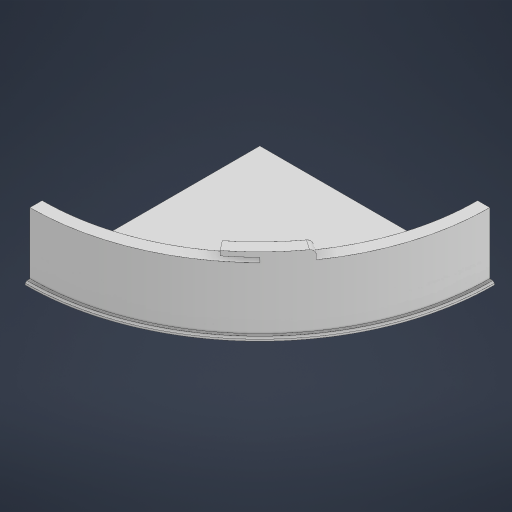
# Autodesk Inventor part: Head_Quad_V1
Saved by Autodesk Inventor 2024 (Build 280153000, 153)
## iProperties
Created: 2025-09-10
Part Number: Head_Quad_V1
Material: Generic
Document SubType Name: Modeling
Designer: kevin
Density: 1 g/cm^3
Appearance: Default
Author: kevin
Autodesk Inventor part; units mm, degrees
ref_plane "YZ Plane" through (0, 0, 0) normal (1, 0, 0) x (0, 1, 0)
ref_plane "XZ Plane" through (0, 0, 0) normal (0, 1, 0) x (-1, 0, 0)
ref_plane "XY Plane" through (0, 0, 0) normal (0, 0, 1) x (1, 0, 0)
sketch "Sketch1" plane through (0, 0, 0) normal (0, 1, 0) x (-1, 0, 0)
  arc A0 (0, 152.4) -> (-152.4, 0) centre (0, 0) ccw
  arc A1 (0, 149.4) -> (-149.4, 0) centre (0, 0) ccw
  line L0 (0, 152.4) -> (0, 0)
  line L1 (0, 152.4) -> (0, 0)
  line L2 (0, 0) -> (-152.4, 0)
  dimension "d0" = 304.8
  dimension "d1" = 3
  constraints: 6 end point, 4 point on circle, 2 centre point, 2 point on line, 1 coincident, 1 collinear, 1 perpendicular, 1 vertical
  measures "d0" diameter of A0
  measures "d1" radial gap between concentric circles of A0 A1
extrude "Extrusion1" add sketch "Sketch1" against normal blind 20
chamfer "Chamfer1" distance 66.675 angle 15 1 edges at (107.7631, -20, 107.7631) measured on face at (67.5943, -20, 75.6381)
sketch "Sketch2" plane through (0, 0, 0) normal (0, 1, 0) x (1, 0, 0)
  line L0 (152.4, 0) -> (0, 0) projected
  line L1 (0, 0) -> (0, -152.4) projected
  arc A0 (0, -152.4) -> (152.4, 0) centre (0, 0) ccw projected
  arc A1 (0, -149.4) -> (149.4, 0) centre (0, 0) ccw projected
  arc A2 (0, -146.4) -> (146.4, 0) centre (0, 0) ccw
  point P0 (146.4, 0)
  point P1 (0, -146.4)
  dimension "d9" = 3
  constraints: 2 point on circle, 1 centre point
  measures "d9" radial gap between concentric circles of A1 A2
extrude "Extrusion3" add sketch "Sketch2" along normal blind 40 contours A1 L1 A2 L0
draft "FaceDraft1" angle -7 pull direction (0, 1, 0) faces at (5.4741, 26.6667, 146.2976) fixed edges at (103.5204, 0, 103.5204)
fillet "Fillet1" radius 3.175 1 edges at (103.5204, 0, 103.5204)
chamfer "Chamfer2" distance 1 angle 45 1 edges at (107.7631, 0, 107.7631)
sketch "Sketch3" plane through (0, 40, 0) normal (0, 1, 0) x (1, 0, 0)
  line L0 (0, -141.4886) -> (0, -149.4) projected
  arc A0 (0, -149.4) -> (149.4, 0) centre (0, 0) ccw projected
  line L1 (149.4, 0) -> (141.4886, 0) projected
  arc A1 (0, -141.4886) -> (141.4886, 0) centre (0, 0) ccw projected
  line L2 (0, 0) -> (105.6418, -105.6418)
  line L3 (0, 0) -> (178.849, 0) construction
  line L4 (0, 0) -> (74.7, -129.3842)
  line L5 (0, 0) -> (178.849, 0) construction
  line L6 (0, 0) -> (122.3813, -85.6923)
  line L7 (0, 0) -> (149.4, 0) construction
  point P0 (115.9007, -81.1545)
  point P1 (100.0476, -100.0476)
  dimension "d17" = 45
  dimension "d18" = 60
  dimension "d19" = 35
  constraints: 12 end point, 3 horizontal, 3 point on circle, 1 equal length
  measures "d17" angle of L2 L3
  measures "d18" angle of L4 L5
  measures "d19" angle of L6 L7
extrude "Extrusion4" add sketch "Sketch3" along normal blind 3 contours A1 L6 A0 L2
sketch "Sketch4" plane through (0, 43, 0) normal (0, 1, 0) x (1, 0, 0)
  line L0 (105.6418, -105.6418) -> (100.0476, -100.0476) projected
  arc A0 (0, -141.4886) -> (100.0476, -100.0476) centre (0, 0) ccw projected
  line L1 (0, -141.4886) -> (0, -149.4) projected
  arc A1 (0, -149.4) -> (105.6418, -105.6418) centre (0, 0) ccw projected
  arc A2 (100.0476, -100.0476) -> (115.9007, -81.1545) centre (0, 0) ccw projected
  line L2 (100.0476, -100.0476) -> (105.6418, -105.6418) projected
  arc A3 (105.6418, -105.6418) -> (122.3813, -85.6923) centre (0, 0) ccw projected
  line L3 (122.3813, -85.6923) -> (115.9007, -81.1545) projected
  line L4 (0, 0) -> (123.1909, -157.6771)
  line L5 (0, 0) -> (200.0951, 0) construction
  point P0 (87.1091, -111.4946)
  point P1 (91.9798, -117.7288)
  dimension "d22" = 52
  constraints: 4 end point, 1 equal length, 1 horizontal
  measures "d22" angle of L4 L5
extrude "Extrusion5" add sketch "Sketch4" along normal blind 3 contours A1 L4 A0 L0 | L0 A2 L3 A3
fillet "Fillet2" radius 3.175 1 edges at (119.141, 46, 83.4234)
sketch "Sketch5" plane through (0, -20, 0) normal (-1, 0, 0) x (0, 0, 1)
  line L0 (151.4, 20) -> (152.4, 19) projected
  line L1 (149.4, 20) -> (151.4, 20) projected
  line L2 (149.4, 20) -> (149.4, 60) projected
  line L3 (141.4886, 60) -> (149.4, 60) projected
  line L4 (145.9626, 23.5619) -> (141.4886, 60) projected
  arc A0 (142.8113, 20) -> (145.9626, 23.5619) centre (142.8113, 23.175) ccw projected
  line L5 (0, 20) -> (142.8113, 20) projected
  line L6 (0, 20) -> (0, 0) projected
  line L7 (85.725, 0) -> (0, 0) projected
  line L8 (152.4, 17.8655) -> (85.725, 0) projected
  line L9 (152.4, 19) -> (152.4, 17.8655) projected
  line L10 (0, 10) -> (123.0455, 10) construction
  circle A1 centre (25, 10) radius 5
  circle A2 centre (85, 10) radius 5
  dimension "d26" = 10
  dimension "d27" = 25
  dimension "d28" = 10
  dimension "d29" = 60
  constraints: 3 point on line, 2 centre point, 2 end point, 1 horizontal, 1 midpoint
  measures "d26" diameter of A1
  measures "d27" distance from line of L6 A1.centre
  measures "d28" diameter of A2
  measures "d29" distance of A2.centre A1.centre
extrude "Extrusion6" add sketch "Sketch5" along normal blind 5 contours A1 | A2
sketch "Sketch6" plane through (0, -20, 0) normal (0, 0, -1) x (-1, 0, 0)
  line L0 (-152.4, 19) -> (-151.4, 20) projected
  line L1 (-152.4, 19) -> (-152.4, 17.8655) projected
  line L2 (-85.725, 0) -> (-152.4, 17.8655) projected
  line L3 (0, 0) -> (-85.725, 0) projected
  line L4 (0, 20) -> (0, 0) projected
  line L5 (-142.8113, 20) -> (0, 20) projected
  arc A0 (-145.9626, 23.5619) -> (-142.8113, 20) centre (-142.8113, 23.175) ccw projected
  line L6 (-145.9626, 23.5619) -> (-141.4886, 60) projected
  line L7 (-149.4, 60) -> (-141.4886, 60) projected
  line L8 (-149.4, 20) -> (-149.4, 60) projected
  line L9 (-151.4, 20) -> (-149.4, 20) projected
  line L10 (0, 10) -> (-123.0455, 10) construction
  circle A1 centre (-25, 10) radius 5.15
  circle A2 centre (-85, 10) radius 5.15
  dimension "d32" = 10.3
  dimension "d33" = 10.3
  dimension "d34" = 25
  dimension "d35" = 60
  constraints: 3 point on line, 2 centre point, 2 end point, 1 horizontal, 1 midpoint
  measures "d32" diameter of A1
  measures "d33" diameter of A2
  measures "d34" distance from line of L4 A1.centre
  measures "d35" distance of A2.centre A1.centre
extrude "Extrusion7" cut sketch "Sketch6" against normal blind 5.3 contours A1 | A2
body "Solid1"
